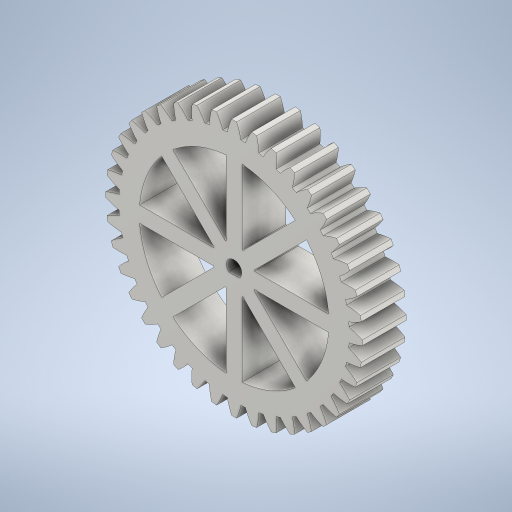
# Autodesk Inventor part: motor_gearMk3
Saved by Autodesk Inventor 2023 (Build 270158000, 158)
## iProperties
CustomPartVersion: 1
Created: 2023-04-03
Part Number: motor_gearMk3
Material: Steel
Document SubType Name: Modeling
Designer: czapa
Categories: <?xml version="1.0" encoding="UTF-16"?> <MemberInstance><Categories><FamilyTemplate><FamilyTemplateParameter ValueType="xs:double" Id="1" ObjectReferenceKey="da_z" ObjectType="kUserParameterObject"/><FamilyTemplateParameter ValueType="xs:double" Id="2" ObjectReferenceKey="da_b" ObjectType="kUserParameterObject"/><FamilyTemplateParameter ValueType="xs:double" Id="3" ObjectReferenceKey="da_beta" ObjectType="kUserParameterObject"/><FamilyTemplateParameter ValueType="xs:double" Id="4" ObjectReferenceKey="da_da" ObjectType="kUserParameterObject"/><FamilyTemplateParameter ValueType="xs:double" Id="5" ObjectReferenceKey="da_aw" ObjectType="kUserParameterObject"/><FamilyTemplateParameter ValueType="xs:string" Id="6" ObjectReferenceKey="EAIAABAAAACIAQAAAAAAAIAAAAAAAAAA" ObjectType="83910656" SubObjectId="SurfaceGeometry"/></FamilyTemplate><ParamToTemplateMap><ParamToTemplate CategoryParameter="//CategoryParameter[@InternalName='046C89C9-8512-4d59-83FE-43B91F4F132A']" TemplateParameter="1"/><ParamToTemplate CategoryParameter="//CategoryParameter[@InternalName='2552DF32-E462-4b46-AEBF-C6C7768E72AC']" TemplateParameter="2"/><ParamToTemplate CategoryParameter="//CategoryParameter[@InternalName='C9EE641D-15FC-4fae-A226-E94C4372FDD7']" TemplateParameter="3"/><ParamToTemplate><ParamToTemplate CategoryParameter="//CategoryParameter[@InternalName='00B6519A-459B-49c7-AD84-2E56D39A5744']" ConstantValue="1.000000"/></ParamToTemplate><ParamToTemplate><ParamToTemplate CategoryParameter="//CategoryParameter[@InternalName='04B31F0E-C7A6-4894-AA32-9629BEFACF47']" ConstantValue="1.000000"/></ParamToTemplate><ParamToTemplate><ParamToTemplate CategoryParameter="//CategoryParameter[@InternalName='43CBEC2E-7847-49e7-A936-2F7889FCB2D9']" ConstantValue="0.250000"/></ParamToTemplate><ParamToTemplate><ParamToTemplate CategoryParameter="//CategoryParameter[@InternalName='B1EFC894-105D-4ebd-86BF-FA20ED196853']" ConstantValue="0.350000"/></ParamToTemplate><ParamToTemplate><ParamToTemplate CategoryParameter="//CategoryParameter[@InternalName='51175063-3D10-4879-93E8-6246FE8B403D']" ConstantValue="2060000000.000000"/></ParamToTemplate><ParamToTemplate><ParamToTemplate CategoryParameter="//CategoryParameter[@InternalName='A3A52E27-4454-46a9-B0BD-C932399B70AF']" ConstantValue="0.300000"/></ParamToTemplate><ParamToTemplate><ParamToTemplate CategoryParameter="//CategoryParameter[@InternalName='91B76062-C214-41d9-B1B9-14D2AB99603D']" ConstantValue="0.200000"/></ParamToTemplate><ParamToTemplate><ParamToTemplate CategoryParameter="//CategoryParameter[@InternalName='374E806E-8B8A-4dda-A9AA-1039D6500AD2']" ConstantValue="5.000000"/></ParamToTemplate><ParamToTemplate><ParamToTemplate CategoryParameter="//CategoryParameter[@InternalName='2D373A89-B862-43d6-8D0B-0CBF12AB9F6C']" ConstantValue="0.349066"/></ParamToTemplate><ParamToTemplate CategoryParameter="//CategoryParameter[@InternalName='37777632-D6A2-4fac-9D53-DB8ACD95C989']" TemplateParameter="4"/><ParamToTemplate CategoryParameter="//CategoryParameter[@InternalName='FD1017F1-B727-4f7e-9707-0F86F1FF9423']" TemplateParameter="5"/><ParamToTemplate><ParamToTemplate CategoryParameter="//CategoryParameter[@InternalName='9E1B4470-B2D3-4ff1-B813-535BB4CDF51A']" ConstantValue="3520000.000000"/></ParamToTemplate><ParamToTemplate><ParamToTemplate CategoryParameter="//CategoryParameter[@InternalName='F8452263-BFF6-458c-9FB1-07C4B99E95CD']" ConstantValue="11400000.000000"/></ParamToTemplate><ParamToTemplate><ParamToTemplate CategoryParameter="//CategoryParameter[@InternalName='3E3BB259-FD49-497f-8171-6EBC954A3479']" ConstantValue="2.000000"/></ParamToTemplate><ParamToTemplate CategoryParameter="//CategoryParameter[@InternalName='27C3BAF2-7550-4e4b-AE2C-0DB134B7D9B7']" TemplateParameter="6"/></ParamToTemplateMap><Category DisplayName="Gear" InternalName="DC85795E-93AB-48d5-8EEE-5A27447B64BD" Mnemonic="Gear"><CategoryParameter DisplayName="z" InternalName="046C89C9-8512-4d59-83FE-43B91F4F132A" Mnemonic="z"/><CategoryParameter DisplayName="b" InternalName="2552DF32-E462-4b46-AEBF-C6C7768E72AC" Mnemonic="b"/><CategoryParameter DisplayName="||b|" InternalName="C9EE641D-15FC-4fae-A226-E94C4372FDD7" Mnemonic="beta"/><CategoryParameter DisplayName="x" InternalName="00B6519A-459B-49c7-AD84-2E56D39A5744" Mnemonic="x"/><CategoryParameter DisplayName="a*" InternalName="04B31F0E-C7A6-4894-AA32-9629BEFACF47" Mnemonic="a"/><CategoryParameter DisplayName="c*" InternalName="43CBEC2E-7847-49e7-A936-2F7889FCB2D9" Mnemonic="c"/><CategoryParameter DisplayName="r|.f|*" InternalName="B1EFC894-105D-4ebd-86BF-FA20ED196853" Mnemonic="rf"/><CategoryParameter DisplayName="E" InternalName="51175063-3D10-4879-93E8-6246FE8B403D" Mnemonic="E"/><CategoryParameter DisplayName="||m|" InternalName="A3A52E27-4454-46a9-B0BD-C932399B70AF" Mnemonic="mi"/><Category DisplayName="SpurGear" InternalName="26C5A22E-A91E-4dfd-A3B3-23CCAFAE1764" Mnemonic="SpurGear"><CategoryParameter DisplayName="m" InternalName="91B76062-C214-41d9-B1B9-14D2AB99603D" Mnemonic="m"/><CategoryParameter DisplayName="P" InternalName="374E806E-8B8A-4dda-A9AA-1039D6500AD2" Mnemonic="PP"/><CategoryParameter DisplayName="||a|" InternalName="2D373A89-B862-43d6-8D0B-0CBF12AB9F6C" Mnemonic="alpha"/><CategoryParameter DisplayName="d|.a|" InternalName="37777632-D6A2-4fac-9D53-DB8ACD95C989" Mnemonic="da"/><CategoryParameter DisplayName="a|.w|" InternalName="FD1017F1-B727-4f7e-9707-0F86F1FF9423" Mnemonic="aw"/><CategoryParameter DisplayName="||s||.Flim|" InternalName="9E1B4470-B2D3-4ff1-B813-535BB4CDF51A" Mnemonic="sFlim"/><CategoryParameter DisplayName="||s||.Hlim|" InternalName="F8452263-BFF6-458c-9FB1-07C4B99E95CD" Mnemonic="sHlim"/><CategoryParameter DisplayName="type" InternalName="3E3BB259-FD49-497f-8171-6EBC954A3479" Mnemonic="type"/><CategoryParameter DisplayName="PitchDiameter" InternalName="27C3BAF2-7550-4e4b-AE2C-0DB134B7D9B7" Mnemonic="IDS_PITCHDIAM"/></Category></Category></Categories></MemberInstance>
Density: 1 g/cm^3
Appearance: Steel
Author: czapa
Autodesk Inventor part; units mm, degrees
ref_plane "YZ Plane" through (0, 0, 0) normal (1, 0, 0) x (0, 1, 0)
ref_plane "XZ Plane" through (0, 0, 0) normal (0, 1, 0) x (-1, 0, 0)
ref_plane "XY Plane" through (0, 0, 0) normal (0, 0, 1) x (1, 0, 0)
sketch "Sketch1" plane through (0, 0, 0) normal (0, 0, 1) x (1, 0, 0)
  circle A0 centre (0, 0) radius 44
  dimension "d0" = 88
  constraints: 1 centre point
  measures "d0" diameter of A0
extrude "Extrusion1" add sketch "Sketch1" along normal blind 15
ref_plane "Work Plane2" through (0, 0, 7.5) normal (0, 0, 1) x (1, 0, 0)
sketch "Sketch2" plane through (0, 0, 0) normal (0, 0, -1) x (-1, 0, 0)
  circle A0 centre (0, 0) radius 44 projected
  circle A1 centre (0, 0) radius 40
  dimension "d3" = 80
  constraints: 1 centre point, 1 coincident
  measures "d3" diameter of A1
surface extrude "Pitch Diameter" sketch "Sketch2" against normal through all shown no curves A1
ref_plane "Work Plane8" through (0, 0, 0) normal (0.9969173, 0.0784591, 0) x (0, 0, 1)
ref_plane "Work Plane9" through (0, 0, 0) normal (1, 0, 0) x (0, 1, 0)
spur gear teeth "Spur Gear" teeth 40 pitch diameter 80 tip diameter 88 root diameter 79 face width 20 start plane through (0, 0, 0) normal (0, 0, -1) x (-1, 0, 0)
sketch "Sketch3" plane through (0, 0, 15) normal (0, 0, 1) x (1, 0, 0)
  circle A0 centre (0, 0) radius 25
  circle A1 centre (0, 0) radius 2.625
  line L0 (0, 2.625) -> (0, -1.875)
  line L1 (0, -1.875) -> (1.8371, -1.875)
  line L2 (0, -1.875) -> (-1.8371, -1.875)
  line L3 (27.107, -3.5241) -> (24.4874, -5.0366)
  line L4 (27.0959, 3.6717) -> (24.4538, 5.1971)
  line L5 (27.0959, 3.6717) -> (27.107, -3.5241)
  line L6 (26.1969, 7.8059) -> (24.4189, 5.3588)
  line L7 (23.2599, 14.3752) -> (26.1969, 7.8059)
  line L8 (23.2599, 14.3752) -> (20.2258, 14.6941)
  line L9 (20.7571, 17.7863) -> (20.1282, 14.8276)
  line L10 (15.4021, 22.593) -> (20.7571, 17.7863)
  line L11 (15.4021, 22.593) -> (12.5006, 21.6503)
  line L12 (11.7282, 24.6913) -> (12.3571, 21.7325)
  line L13 (4.8811, 26.9044) -> (11.7282, 24.6913)
  line L14 (4.8811, 26.9044) -> (2.6139, 24.863)
  line L15 (0.6714, 27.3269) -> (2.4493, 24.8797)
  line L16 (-6.4839, 26.5637) -> (0.6714, 27.3269)
  line L17 (-6.4839, 26.5637) -> (-7.7248, 23.7766)
  line L18 (-10.5015, 25.2374) -> (-7.8819, 23.725)
  line L19 (-16.7277, 21.6299) -> (-10.5015, 25.2374)
  line L20 (-16.7277, 21.6299) -> (-16.7277, 18.5791)
  line L21 (-19.8586, 18.7842) -> (-16.8503, 18.468)
  line L22 (-24.0792, 12.9561) -> (-19.8586, 18.7842)
  line L23 (-24.0792, 12.9561) -> (-22.8383, 10.1691)
  line L24 (-25.7819, 9.083) -> (-22.9051, 10.0177)
  line L25 (-27.2672, 2.0421) -> (-25.7819, 9.083)
  line L26 (-27.2672, 2.0421) -> (-25, 0.0007)
  line L27 (-27.2473, -2.1887) -> (-24.9995, -0.1647)
  line L28 (-25.7404, -9.225) -> (-27.2473, -2.1887)
  line L29 (-25.7404, -9.225) -> (-22.8389, -10.1678)
  line L30 (-24.0015, -13.082) -> (-22.7711, -10.3187)
  line L31 (-19.7629, -18.897) -> (-24.0015, -13.082)
  line L32 (-19.7629, -18.897) -> (-16.7288, -18.5781)
  line L33 (-16.6055, -21.7133) -> (-16.6055, -18.6884)
  line L34 (-10.3682, -25.3016) -> (-16.6055, -21.7133)
  line L35 (-10.3682, -25.3016) -> (-7.7261, -23.7762)
  line L36 (-6.3383, -26.5901) -> (-7.5686, -23.8268)
  line L37 (0.8193, -27.3313) -> (-6.3383, -26.5901)
  line L38 (0.8193, -27.3313) -> (2.6125, -24.8631)
  line L39 (5.0249, -26.8693) -> (2.777, -24.8453)
  line L40 (11.8651, -24.6351) -> (5.0249, -26.8693)
  line L41 (11.8651, -24.6351) -> (12.4994, -21.651)
  line L42 (15.5192, -22.5025) -> (12.6424, -21.5678)
  line L43 (20.8593, -17.6793) -> (15.5192, -22.5025)
  line L44 (20.8593, -17.6793) -> (20.225, -14.6952)
  line L45 (23.3301, -14.2449) -> (20.3218, -14.5611)
  line L46 (26.2468, -7.6666) -> (23.3301, -14.2449)
  line L47 (26.2468, -7.6666) -> (24.4535, -5.1985)
  point P0 (20.2258, 14.6941)
  point P1 (24.4189, 5.3588)
  point P2 (12.5006, 21.6503)
  point P3 (20.1282, 14.8276)
  point P4 (2.6139, 24.863)
  point P5 (12.3571, 21.7325)
  point P6 (-7.7248, 23.7766)
  point P7 (2.4493, 24.8797)
  point P8 (-16.7277, 18.5791)
  point P9 (-7.8819, 23.725)
  point P10 (-22.8383, 10.1691)
  point P11 (-16.8503, 18.468)
  point P12 (-25, 0.0007)
  point P13 (-22.9051, 10.0177)
  point P14 (-22.8389, -10.1678)
  point P15 (-24.9995, -0.1647)
  point P16 (-16.7288, -18.5781)
  point P17 (-22.7711, -10.3187)
  point P18 (-7.7261, -23.7762)
  point P19 (-16.6055, -18.6884)
  point P20 (2.6125, -24.8631)
  point P21 (-7.5686, -23.8268)
  point P22 (12.4994, -21.651)
  point P23 (2.777, -24.8453)
  point P24 (20.225, -14.6952)
  point P25 (12.6424, -21.5678)
  point P26 (24.4535, -5.1985)
  point P27 (20.3218, -14.5611)
  dimension "d51" = 50
  dimension "d52" = 5.25
  dimension "d53" = 4.5
  dimension "d54" = 360
  constraints: 96 end point, 5 point on circle, 2 centre point, 2 coincident, 1 horizontal, 1 point on line, 1 vertical, 106 other
  measures "d51" diameter of A0
  measures "d52" diameter of A1
  measures "d53" distance of L0.start L0.end
extrude "Extrusion2" cut sketch "Sketch3" against normal blind 15 contours A1 L1 L0 | L0 L2 A1
sketch "Sketch4" plane through (0, 0, 15) normal (0, 0, 1) x (1, 0, 0)
  arc A0 (2.3254, -39.4315) -> (3.8717, -39.3098) centre (0, 0) ccw projected
  circle A1 centre (0, 0) radius 39.5
  circle A2 centre (0, 0) radius 32.5
  line L0 (0, 0) -> (25, 0) construction
  circle A3 centre (0, 0) radius 7.5
  line L1 (0, 7.5) -> (0, 32.5)
  line L2 (2.7208, 6.9891) -> (2.7208, 32.3859)
  line L3 (-2.7208, 6.9891) -> (-2.7208, 32.3859)
  line L4 (-3.0181, 6.8659) -> (-20.9764, 24.8242)
  line L5 (-6.8659, 3.0181) -> (-24.8242, 20.9764)
  line L6 (-6.9891, 2.7208) -> (-32.3859, 2.7208)
  line L7 (-6.9891, -2.7208) -> (-32.3859, -2.7208)
  line L8 (-6.8659, -3.0181) -> (-24.8242, -20.9764)
  line L9 (-3.0181, -6.8659) -> (-20.9764, -24.8242)
  line L10 (-2.7208, -6.9891) -> (-2.7208, -32.3859)
  line L11 (2.7208, -6.9891) -> (2.7208, -32.3859)
  line L12 (3.0181, -6.8659) -> (20.9764, -24.8242)
  line L13 (6.8659, -3.0181) -> (24.8242, -20.9764)
  line L14 (6.9891, -2.7208) -> (32.3859, -2.7208)
  line L15 (6.9891, 2.7208) -> (32.3859, 2.7208)
  line L16 (6.8659, 3.0181) -> (24.8242, 20.9764)
  line L17 (3.0181, 6.8659) -> (20.9764, 24.8242)
  point P0 (-32.3859, -2.7208)
  dimension "d57" = 65
  dimension "d59" = 15
  dimension "d62" = 360
  constraints: 36 end point, 4 point on circle, 3 coincident, 2 centre point, 2 symmetric about line, 1 horizontal, 1 parallel, 1 vertical, 52 other
  measures "d57" diameter of A2
  measures "d59" diameter of A3
extrude "Extrusion3" cut sketch "Sketch4" against normal blind 15 contours L15 A3 L16 A2 | A2 L13 A3 L14 | L17 A3 L2 A2 | A2 L11 A3 L12 | A2 L9 A3 L10 | L3 A3 L4 A2 | A2 L7 A3 L8 | L5 A3 L6 A2
equation "\"d0\" = da_da"
equation "\"d3\" = da_d"
equation "\"da_da\" = 88"
equation "\"da_d\" = 80"
body "Solid1"
body "Srf1"
